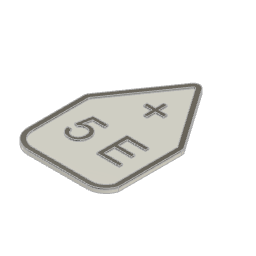
_Pointed Marker Single +.05bee052-56c8-47a5-914a-778622fd047e (Autodesk Fusion 360 design; units mm, degrees)
Autodesk Fusion 360 part; units mm, degrees
sketch "Sketch1" plane through (0, 0, 0) normal (0, 0, 1) x (1, 0, 0)
  line L0 (0, 50.8) -> (0, 0)
  arc A0 (-31.7281, 6.3281) -> (-25.4, 0) centre (-25.4, 6.3281) ccw
  line L1 (-25.4, 0) -> (-15.875, 0)
  line L2 (-31.7281, 25.3781) -> (-31.7281, 6.3281)
  line L3 (-31.7281, 25.3781) -> (-15.7092, 48.2556)
  line L4 (-6.0183, 0) -> (-15.5433, 0)
  line L5 (0.3098, 25.3781) -> (-15.7092, 48.2556)
  arc A1 (-6.0183, 0) -> (0.3098, 6.3281) centre (-6.0183, 6.3281) ccw
  line L6 (0.3098, 25.3781) -> (0.3098, 6.3281)
  line L7 (-15.875, 0) -> (-15.5433, 0)
  dimension "d4" = 50.8
  dimension "d12" = 19.05
  constraint vertical L0
  constraint coincident L0.end origin
  constraint tangent A0 L1
  constraint vertical L2
  constraint parallel L4 L7
  measures "d4" distance of L0.end L0.start
  measures "d12" distance of A0.start L2.start
extrude "Extrude1" add sketch "Sketch1" along normal blind 1 contours L0 A0 L1 L2 L3 L4 L5 A1 L7 makes body 1
fillet "Fillet1" radius 2 3 edges at (0, 25.8206, 0.5) (-31.7281, 25.3781, 0.5) (-15.7092, 48.2556, 0.5) on bodies 1
sketch "Sketch2" plane through (0, 0, 1) normal (0, 0, 1) x (-1, 0, 0)
  arc A0 (14.0709, -45.9158) -> (17.3475, -45.9158) centre (15.7092, -44.7687) ccw
  line L0 (17.3475, -45.9158) -> (31.3664, -25.8947)
  arc A1 (31.3664, -25.8947) -> (31.7281, -24.7475) centre (29.7281, -24.7475) ccw
  line L1 (31.7281, -24.7475) -> (31.7281, -6.3281)
  arc A2 (31.7281, -6.3281) -> (25.4, 0) centre (25.4, -6.3281) ccw
  line L2 (25.4, 0) -> (6.0183, 0)
  arc A3 (6.0183, 0) -> (0, -4.3724) centre (6.0183, -6.3281) ccw
  line L3 (0, -4.3724) -> (0, -25.19)
  arc A4 (0, -25.19) -> (0.3617, -26.3371) centre (2, -25.19) ccw
  line L4 (0.3617, -26.3371) -> (14.0709, -45.9158)
  line L5 (16.1187, -45.0555) -> (30.1377, -25.0343)
  arc A5 (30.1377, -25.0343) -> (30.2281, -24.7475) centre (29.7281, -24.7475) ccw
  line L6 (30.2281, -24.7475) -> (30.2281, -6.3281)
  arc A6 (30.2281, -6.3281) -> (25.4, -1.5) centre (25.4, -6.3281) ccw
  line L7 (25.4, -1.5) -> (6.0183, -1.5)
  arc A7 (6.0183, -1.5) -> (1.5, -4.6265) centre (6.0183, -6.3281) ccw
  line L8 (1.5, -4.6265) -> (1.5, -25.19)
  arc A8 (1.5, -25.19) -> (1.5904, -25.4768) centre (2, -25.19) ccw
  line L9 (1.5904, -25.4768) -> (15.2996, -45.0555)
  arc A9 (15.2996, -45.0555) -> (16.1187, -45.0555) centre (15.7092, -44.7687) ccw
  line L10 (25.6864, -13.7884) -> (3.6261, -13.7884) construction
  line L11 (3.6261, -13.7884) -> (3.6261, -25.3842) construction
  line L12 (3.6261, -25.3842) -> (25.6864, -25.3842) construction
  line L13 (25.6864, -25.3842) -> (25.6864, -13.7884) construction
  dimension "d18" = -1.5
  dimension "d19" = 10.0076
copy_body "Body->Comp1" bodies 1 removing the originals makes body 2 in component "Arrow Base"
sketch "Sketch3" plane through (0, 0, 1) normal (0, 0, 1) x (-1, 0, 0)
  arc A0 (14.0709, -45.9158) -> (17.3475, -45.9158) centre (15.7092, -44.7687) ccw
  line L0 (17.3475, -45.9158) -> (31.3664, -25.8947)
  arc A1 (31.3664, -25.8947) -> (31.7281, -24.7475) centre (29.7281, -24.7475) ccw
  line L1 (31.7281, -24.7475) -> (31.7281, -6.3281)
  arc A2 (31.7281, -6.3281) -> (25.4, 0) centre (25.4, -6.3281) ccw
  line L2 (25.4, 0) -> (6.0183, 0)
  arc A3 (6.0183, 0) -> (0, -4.3724) centre (6.0183, -6.3281) ccw
  line L3 (0, -4.3724) -> (0, -25.19)
  arc A4 (0, -25.19) -> (0.3617, -26.3371) centre (2, -25.19) ccw
  line L4 (0.3617, -26.3371) -> (14.0709, -45.9158)
  line L5 (16.1187, -45.0555) -> (30.1377, -25.0343)
  arc A5 (30.1377, -25.0343) -> (30.2281, -24.7475) centre (29.7281, -24.7475) ccw
  line L6 (30.2281, -24.7475) -> (30.2281, -6.3281)
  arc A6 (30.2281, -6.3281) -> (25.4, -1.5) centre (25.4, -6.3281) ccw
  line L7 (25.4, -1.5) -> (6.0183, -1.5)
  arc A7 (6.0183, -1.5) -> (1.5, -4.6265) centre (6.0183, -6.3281) ccw
  line L8 (1.5, -4.6265) -> (1.5, -25.19)
  arc A8 (1.5, -25.19) -> (1.5904, -25.4768) centre (2, -25.19) ccw
  line L9 (1.5904, -25.4768) -> (15.2996, -45.0555)
  arc A9 (15.2996, -45.0555) -> (16.1187, -45.0555) centre (15.7092, -44.7687) ccw
  line L10 (29.7281, -6.1121) -> (1.5, -6.1121) construction
  line L11 (1.5, -6.1121) -> (1.5, -24.7475) construction
  line L12 (1.5, -24.7475) -> (29.7281, -24.7475) construction
  line L13 (29.7281, -24.7475) -> (29.7281, -6.1121) construction
  line L14 (22.698, -27.7932) -> (8.8204, -27.7932) construction
  line L15 (8.8204, -27.7932) -> (8.8204, -35.5954) construction
  line L16 (8.8204, -35.5954) -> (22.698, -35.5954) construction
  line L17 (22.698, -35.5954) -> (22.698, -27.7932) construction
  dimension "d26" = -1.5
  dimension "d37" = 10.0076
  dimension "d41" = 10.0076
  text T0 "5 E" font "Arial" height 10.0076 align centre middle in box 28.2281 x 18.6354 at (29.7281, -6.1121) x (-1, 0) y (0, -1) spacing 1 kerned
  text T1 "+\n" font "Arial" height 10.0076 align centre top in box 13.8776 x 7.8022 at (22.698, -27.7932) x (-1, 0) y (0, -1) spacing 1 kerned
extrude "Extrude1'" add sketch "Sketch3" sketch "Sketch3" along normal blind 0.5 separate body of sketch 2 text T1 T0 makes body 3 at (-15.5658, 29.8953, 1) makes body 4 at (-21.6109, 38.9553, 1) makes body 5 at (-22.2665, 19.9057, 1) makes body 6 at (-12.8141, 15.291, 1) in component "Component"
component "Letters" placed x (1, 0, 0) y (0, 1, 0) z (0, 0, 1) at (0, 0, 0)
component "Component" placed x (1, 0, 0) y (0, 1, 0) z (0, 0, 1) at (0, 0, 0)
component "Arrow Base" placed x (1, 0, 0) y (0, 1, 0) z (0, 0, 1) at (0, 0, 0)
equation "Num = 3" comment "5 E"
equation "Num2 = 4"
equation "Ɠ = "
equation "Ɛ = "
equation "ƍ = "
equation "Ɗ = "
equation "Ƈ = "
equation "Ƅ = "
equation "Ɓ = "
equation "Ɩ = "
equation "Ƣ = "
equation "Ɵ = "
equation "Ɯ = "
equation "ƙ = "
equation "ƥ = "
equation "Ż = "
equation "Ÿ = "
equation "ŵ = "
equation "Ų = "
equation "ů = "
equation "Ŭ = "
equation "ũ = "
equation "Ŧ = "
equation "ž = "
equation "ƾ = "
equation "ƻ = "
equation "Ƹ = "
equation "Ƶ = "
equation "Ʋ = "
equation "Ư = "
equation "Ƭ = "
equation "Ʃ = "
equation "Ʀ = "
equation "ƣ = "
equation "Ơ = "
equation "ǁ = "
equation "ǜ = "
equation "Ǚ = "
equation "ǖ = "
equation "Ǔ = "
equation "ǐ = "
equation "Ǎ = "
equation "Ǌ = "
equation "Ǉ = "
equation "Ǆ = "
equation "ǟ = "
equation "ƚ = "
equation "Ɨ = "
equation "Ɣ = "
equation "Ƒ = "
equation "Ǝ = "
equation "Ƌ = "
equation "ƈ = "
equation "ƅ = "
equation "Ɲ = "
equation "ǻ = "
equation "Ǹ = "
equation "ǵ = "
equation "ǲ = "
equation "ǯ = "
equation "Ǭ = "
equation "ǩ = "
equation "Ǧ = "
equation "ǣ = "
equation "Ǡ = "
equation "ǝ = "
equation "ǚ = "
equation "Ǘ = "
equation "ǔ = "
equation "Ǒ = "
equation "ǎ = "
equation "ǋ = "
equation "ǈ = "
equation "ǅ = "
equation "ǂ = "
equation "ƿ = "
equation "Ǿ = "
equation "ƹ = "
equation "ƶ = "
equation "Ƴ = "
equation "ư = "
equation "ƭ = "
equation "ƪ = "
equation "Ƨ = "
equation "Ƥ = "
equation "Ƽ = "
equation "ǡ = "
equation "Ǟ = "
equation "Ǜ = "
equation "ǘ = "
equation "Ǖ = "
equation "ǒ = "
equation "Ǐ = "
equation "ǌ = "
equation "ǉ = "
equation "ǆ = "
equation "ǃ = "
equation "Ǥ = "
equation "ț = "
equation "Ș = "
equation "ȕ = "
equation "Ȓ = "
equation "ȏ = "
equation "Ȍ = "
equation "ȉ = "
equation "Ȇ = "
equation "ȃ = "
equation "Ȁ = "
equation "ǽ = "
equation "Ȟ = "
equation "Ƿ = "
equation "Ǵ = "
equation "Ǳ = "
equation "Ǯ = "
equation "ǫ = "
equation "Ǩ = "
equation "ǥ = "
equation "Ǣ = "
equation "Ǻ = "
equation "ȟ = "
equation "Ȝ = "
equation "ș = "
equation "Ȗ = "
equation "ȓ = "
equation "Ȑ = "
equation "ȍ = "
equation "Ȋ = "
equation "ȇ = "
equation "Ȅ = "
equation "ȁ = "
equation "Ȣ = "
equation "ɍ = "
equation "Ɋ = "
equation "ɇ = "
equation "Ʉ = "
equation "Ɂ = "
equation "Ⱦ = "
equation "Ȼ = "
equation "ɐ = "
equation "ɜ = "
equation "ə = "
equation "ɖ = "
equation "ɓ = "
equation "ɟ = "
equation "ȵ = "
equation "Ȳ = "
equation "ȯ = "
equation "Ȭ = "
equation "ȩ = "
equation "Ȧ = "
equation "ȣ = "
equation "Ƞ = "
equation "ȸ = "
equation "ɸ = "
equation "ɵ = "
equation "ɲ = "
equation "ɯ = "
equation "ɬ = "
equation "ɩ = "
equation "ɦ = "
equation "ɣ = "
equation "ɠ = "
equation "ɝ = "
equation "ɚ = "
equation "ɻ = "
equation "ɔ = "
equation "ɑ = "
equation "Ɏ = "
equation "ɋ = "
equation "Ɉ = "
equation "Ʌ = "
equation "ɂ = "
equation "ȿ = "
equation "ɗ = "
equation "ʝ = "
equation "ʚ = "
equation "ʗ = "
equation "ʔ = "
equation "ʑ = "
equation "ʎ = "
equation "ʋ = "
equation "ʈ = "
equation "ʅ = "
equation "ʂ = "
equation "ɿ = "
equation "ɼ = "
equation "ɹ = "
equation "ʠ = "
equation "ː = "
equation "ˍ = "
equation "ˊ = "
equation "ˇ = "
equation "ˁ = "
equation "ʾ = "
equation "ʸ = "
equation "ʵ = "
equation "ʲ = "
equation "ʯ = "
equation "ʬ = "
equation "ʩ = "
equation "ʦ = "
equation "ʣ = "
equation "ʻ = "
equation "ɳ = "
equation "ɰ = "
equation "ɭ = "
equation "ɪ = "
equation "ɧ = "
equation "ɤ = "
equation "ɡ = "
equation "ɞ = "
equation "ɶ = "
equation "ƃ = "
equation "ű = "
equation "Ŵ = "
equation "Ŷ = "
equation "Ź = "
equation "ƀ = "
equation "ğ = "
equation "Ġ = "
equation "ċ = "
equation "č = "
equation "Đ = "
equation "Ē = "
equation "ĕ = "
equation "ė = "
equation "Ě = "
equation "Ĝ = "
equation "ơ = "
equation "ƨ = "
equation "ƫ = "
equation "Ə = "
equation "ƒ = "
equation "ĸ = "
equation "Ĺ = "
equation "Ĥ = "
equation "Ħ = "
equation "ĩ = "
equation "ī = "
equation "Į = "
equation "İ = "
equation "ĳ = "
equation "ĵ = "
equation "Ū = "
equation "ū = "
equation "Ŗ = "
equation "Ř = "
equation "ś = "
equation "ŝ = "
equation "Š = "
equation "Ţ = "
equation "ť = "
equation "ŧ = "
equation "ő = "
equation "Œ = "
equation "Ľ = "
equation "Ŀ = "
equation "ł = "
equation "ń = "
equation "Ň = "
equation "ŉ = "
equation "Ō = "
equation "Ŏ = "
equation "ƺ = "
equation "Ʒ = "
equation "ƴ = "
equation "Ʊ = "
equation "Ʈ = "
equation "ɴ = "
equation "ɱ = "
equation "ɮ = "
equation "ɫ = "
equation "ɨ = "
equation "ɥ = "
equation "ɺ = "
equation "ʆ = "
equation "ˮ = "
equation "ʜ = "
equation "ʙ = "
equation "ʖ = "
equation "ʓ = "
equation "ʐ = "
equation "ʍ = "
equation "ʊ = "
equation "ʇ = "
equation "ȳ = "
equation "Ȱ = "
equation "ȭ = "
equation "Ȫ = "
equation "ȧ = "
equation "Ȥ = "
equation "Ǫ = "
equation "ǧ = "
equation "Ȃ = "
equation "ǿ = "
equation "Ǽ = "
equation "ȅ = "
equation "ȑ = "
equation "Ȏ = "
equation "ȋ = "
equation "Ȉ = "
equation "ȝ = "
equation "ʞ = "
equation "ʛ = "
equation "ʘ = "
equation "ʕ = "
equation "ʒ = "
equation "ʏ = "
equation "ʌ = "
equation "ʉ = "
equation "ʼ = "
equation "ʹ = "
equation "ʶ = "
equation "ʳ = "
equation "ʰ = "
equation "ʭ = "
equation "ʪ = "
equation "ˑ = "
equation "ˎ = "
equation "ˋ = "
equation "ˈ = "
equation "ˣ = "
equation "ˠ = "
equation "ȴ = "
equation "ȱ = "
equation "Ȯ = "
equation "ȫ = "
equation "Ȩ = "
equation "ȥ = "
equation "ʷ = "
equation "ʴ = "
equation "ʱ = "
equation "ʮ = "
equation "ʫ = "
